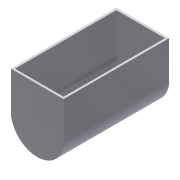
# Autodesk Inventor part: Composter
Saved by Autodesk Inventor 2019 (Build 230136000, 136)
## iProperties
Created: 2020-02-29
Part Number: Composter
Material: Generic
Document SubType Name: Modeling
Designer: stef_
Density: 1 g/cm^3
Appearance: PVC - White
Author: stef_
Autodesk Inventor part; units mm, degrees
ref_plane "YZ Plane" through (0, 0, 0) normal (1, 0, 0) x (0, 1, 0)
ref_plane "XZ Plane" through (0, 0, 0) normal (0, 1, 0) x (-1, 0, 0)
ref_plane "XY Plane" through (0, 0, 0) normal (0, 0, 1) x (1, 0, 0)
sketch "Sketch1" plane through (0, 0, 0) normal (0, 0, 1) x (1, 0, 0)
  line L0 (-216.5289, 82.2753) -> (-216.5289, 432.2753)
  line L1 (-216.5289, 432.2753) -> (283.4711, 432.2753)
  line L2 (283.4711, 432.2753) -> (283.4711, 82.2753)
  arc A0 (-216.5289, 82.2753) -> (283.4711, 82.2753) centre (33.4711, 82.2753) ccw
  point P0 (0, 0)
  dimension "d0" = 500
  dimension "d1" = 250
  dimension "d2" = 350
  constraints: 6 end point, 2 perpendicular, 2 point on circle, 1 centre point, 1 parallel, 1 vertical
  measures "d0" distance of L0.end L1.end
  measures "d1" radius of A0
  measures "d2" distance of L1.end L2.end
extrude "Extrusion1" add sketch "Sketch1" against normal blind 1000
shell "Shell1" thickness 20 removed faces 1 at (-49.8623, 432.2753, -333.3333)
ref_plane "Work Plane1" through (-216.5289, -262.4747, 0) normal (0, 1, 0) x (-1, 0, 0)
sketch "Sketch2" plane through (-216.5289, -262.4747, 0) normal (0, 1, 0) x (-1, 0, 0)
  point P0 (-216.5289, 0)
sketch "Sketch3" plane through (-216.5289, -262.4747, 0) normal (0, 1, 0) x (-1, 0, 0)
  line L0 (-110, -915) -> (-30, -915)
  line L1 (-30, -915) -> (-30, -835)
  line L2 (-30, -835) -> (-110, -835)
  line L3 (-110, -835) -> (-110, -915)
  line L4 (-390, -915) -> (-470, -915)
  line L5 (-470, -915) -> (-470, -835)
  line L6 (-470, -835) -> (-390, -835)
  line L7 (-390, -835) -> (-390, -915)
  line L8 (-500, 0) -> (-500, -1000) projected
  line L9 (0, 0) -> (0, -1000) projected
  line L10 (-500, -1000) -> (0, -1000) projected
  line L11 (0, 0) -> (0, -1000) projected
  line L12 (0, -500) -> (-564.0368, -500)
  line L13 (-110, -85) -> (-30, -85)
  line L14 (-30, -85) -> (-30, -165)
  line L15 (-110, -165) -> (-110, -85)
  line L16 (-390, -85) -> (-470, -85)
  line L17 (-470, -85) -> (-470, -165)
  line L18 (-470, -165) -> (-390, -165)
  line L19 (-390, -165) -> (-390, -85)
  line L20 (-110, -165) -> (-30, -165)
  point P0 (-216.5289, 0)
  dimension "d6" = 80
  dimension "d7" = 80
  dimension "d8" = 30
  dimension "d10" = 30
  dimension "d11" = 85
  constraints: 34 end point, 8 symmetric about line, 4 horizontal, 4 parallel, 2 equal length, 2 perpendicular, 1 midpoint, 1 point on line
  measures "d6" distance of L5.end L6.end
  measures "d7" distance of L4.end L5.end
  measures "d8" distance between parallel lines of L8 L5
  measures "d10" distance between parallel lines of L9 L1
  measures "d11" distance between parallel lines of L10 L4
extrude "Extrusion2" add sketch "Sketch3" along normal up to next contours L3 L2 L1 L0 | L4 L5 L6 L7 | L13 L14 L20 L15 | L19 L18 L17 L16
sketch "Sketch4" plane through (-216.5289, 432.2753, 0) normal (0, 1, 0) x (1, 0, 0)
  line L0 (14.5, 14.5) -> (485.5, 14.5)
  line L1 (485.5, 14.5) -> (485.5, 985.5)
  line L2 (485.5, 985.5) -> (14.5, 985.5)
  line L3 (14.5, 985.5) -> (14.5, 14.5)
  line L4 (480, 980) -> (480, 20) projected
  line L5 (480, 20) -> (20, 20) projected
  line L6 (20, 20) -> (20, 980) projected
  line L7 (20, 980) -> (480, 980) projected
  point P0 (216.5289, 0)
  dimension "d14" = 5.5
  dimension "d15" = 5.5
  dimension "d16" = 5.5
  dimension "d17" = 5.5
  constraints: 8 end point, 2 parallel, 1 horizontal, 1 perpendicular
  measures "d14" distance between parallel lines of L4 L1
  measures "d15" distance between parallel lines of L5 L0
  measures "d16" distance between parallel lines of L6 L3
  measures "d17" distance between parallel lines of L7 L2
extrude "Extrusion3" cut sketch "Sketch4" against normal blind 30
body "Solid1"
